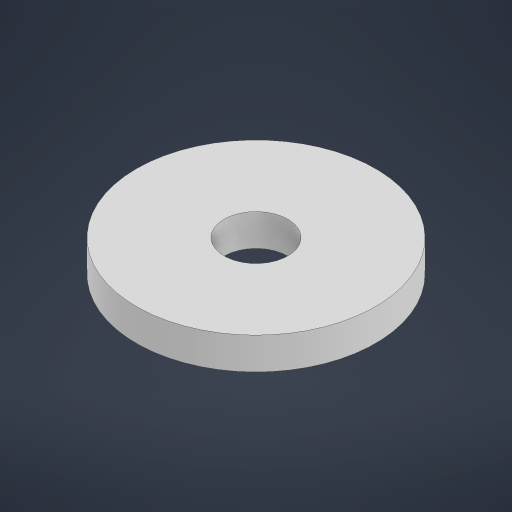
# Autodesk Inventor part: load_bearing
Saved by Autodesk Inventor 2024 (Build 280153000, 153)
## iProperties
Created: 2023-05-23
Part Number: load_bearing
Material: Generic
Document SubType Name: Modeling
Designer: aasmu
Density: 1 g/cm^3
Appearance: Default
load_bearing_ID: 4.000 mm
load_bearing_OD: 15.000 mm
load_bearing_W: 2.000 mm
Author: aasmu
Autodesk Inventor part; units mm, degrees
ref_plane "YZ Plane" through (0, 0, 0) normal (1, 0, 0) x (0, 1, 0)
ref_plane "XZ Plane" through (0, 0, 0) normal (0, 1, 0) x (-1, 0, 0)
ref_plane "XY Plane" through (0, 0, 0) normal (0, 0, 1) x (1, 0, 0)
sketch "Sketch1" plane through (0, 0, 0) normal (0, 1, 0) x (-1, 0, 0)
  circle A0 centre (0, 0) radius 2
  circle A1 centre (0, 0) radius 7.5
  dimension "load_bearing_ID" = 4
  dimension "load_bearing_OD" = 15
  constraints: 2 centre point, 2 coincident
  measures "load_bearing_ID" diameter of A0
  measures "load_bearing_OD" diameter of A1
extrude "Extrusion1" add sketch "Sketch1" along normal blind 2
equation "\"load_bearing_ID\" = cabel_roller_ID"
equation "\"d2\" = load_bearing_W"
equation "\"load_bearing_W\" = 2"
equation "\"cabel_roller_ID\" = 4"
body "Solid1"
